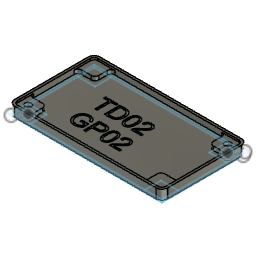
PDP_ETUDIANTS_3D_TD02_GP02 (Autodesk Fusion 360 archive; units mm, degrees)
design "Boitier Bas"
Autodesk Fusion 360 part; units mm, degrees
sketch "Sketch1" plane through (0, 0, 0) normal (0, 0, 1) x (1, 0, 0)
  line L0 (-40, 30) -> (39, 30)
  line L1 (39, 30) -> (39, -14)
  line L2 (39, -14) -> (-40, -14)
  line L3 (39, 30) -> (39, 28)
  line L4 (-40, 30) -> (-40, -14)
  circle A0 centre (-35, -9) radius 1.6
  circle A1 centre (34, 25) radius 1.6
  line L5 (39, 30) -> (37.8, 30)
  line L6 (-40, -14) -> (-38.8, -14)
  line L7 (37.8, 28.8) -> (-38.8, 28.8)
  line L8 (-38.8, 28.8) -> (-38.8, -12.8)
  line L9 (-38.8, -12.8) -> (37.8, -12.8)
  line L10 (37.8, -12.8) -> (37.8, 28.8)
  line L11 (-30.0372, -12.8) -> (-30.0372, -4.5)
  line L12 (-30.0372, -4.5) -> (-38.8, -4.5)
  line L13 (-30.037, 28.8) -> (-30.037, 20.5)
  line L14 (-30.037, 20.5) -> (-38.8, 20.5)
  line L15 (37.8, 20.5) -> (29.037, 20.5)
  line L16 (29.037, 20.5) -> (29.037, 28.8)
  line L17 (29.037, -12.8) -> (29.037, -4.5)
  line L18 (29.037, -4.5) -> (37.8, -4.5)
  line L19 (-31.8769, -9.5739) -> (-32.9414, -6.5822)
  line L20 (-32.9414, -6.5822) -> (-36.0646, -6.0083)
  line L21 (-36.0646, -6.0083) -> (-38.1231, -8.4261)
  line L22 (-38.1231, -8.4261) -> (-37.0586, -11.4178)
  line L23 (-37.0586, -11.4178) -> (-33.9354, -11.9917)
  line L24 (-33.9354, -11.9917) -> (-31.8769, -9.5739)
  line L25 (30.8264, 24.8932) -> (32.5057, 22.1982)
  line L26 (32.5057, 22.1982) -> (35.6793, 22.305)
  line L27 (35.6793, 22.305) -> (37.1736, 25.1068)
  line L28 (37.1736, 25.1068) -> (35.4943, 27.8018)
  line L29 (35.4943, 27.8018) -> (32.3207, 27.695)
  line L30 (32.3207, 27.695) -> (30.8264, 24.8932)
  point P0 (-35, -9)
  point P1 (34, 25)
  dimension "d1" = 79
  dimension "d2" = 44
  dimension "d6" = 3.2
  dimension "d8" = 3.2
  dimension "d32" = 8.3
  dimension "d33" = 8.763
  dimension "d35" = 8.763
  dimension "d36" = 8.763
  dimension "d37" = 8.3
  dimension "d38" = 8.3
  dimension "d39" = 8.3
  dimension "d65" = 2.75
  dimension "d70" = 2.75
  constraint horizontal L0
  constraint vertical L1
  constraint horizontal L2
  constraint perpendicular L0 L3
  constraint perpendicular L2 L4
  constraint perpendicular L3 L5
  constraint perpendicular L4 L6
  constraint horizontal L7
  constraint vertical L8
  constraint horizontal L9
  constraint vertical L10
  constraint coincident L9 L11.start
  constraint perpendicular L9 L11
  constraint coincident L8 L12.end
  constraint perpendicular L8 L12
  constraint coincident L7 L13.start
  constraint perpendicular L7 L13
  constraint coincident L8 L14.end
  constraint perpendicular L8 L14
  constraint coincident L10 L15.start
  constraint perpendicular L10 L15
  constraint coincident L7 L16.end
  constraint perpendicular L7 L16
  constraint coincident L9 L17.start
  constraint perpendicular L9 L17
  constraint coincident L10 L18.end
  constraint perpendicular L10 L18
  constraint coincident P0 A0.centre
  constraint coincident P1 A1.centre
  measures "d1" distance of L0.start L0.end
  measures "d2" distance of L0.start L2.end
  measures "d6" diameter of A0
  measures "d8" diameter of A1
  measures "d32" distance of L17.start L17.end
  measures "d33" distance of L13.end L14.end
  measures "d35" distance of L17.end L18.end
  measures "d36" distance of L15.start L15.end
  measures "d37" distance of L15.end L16.end
  measures "d38" distance of L11.start L11.end
  measures "d39" distance of L13.start L13.end
  measures "d65" distance of P0 L24
  measures "d70" distance of P1 L30
extrude "Extrude3" add sketch "Sketch1" along normal blind 5 contours L0 L1 L2 L3 L4 L5 L6
extrude "Extrude4" add sketch "Sketch1" along normal blind 4 contours L9 L10 L17 L18
extrude "Extrude5" add sketch "Sketch1" along normal blind 4 contours L7 L8 L13 L14
extrude "Extrude6" add sketch "Sketch1" along normal blind 4 contours A0 | L8 L9 L11 L12 | L19 L20 L21 L22 L23 L24
extrude "Extrude7" add sketch "Sketch1" along normal blind 4 contours A1 | L7 L10 L15 L16 | L25 L26 L27 L28 L29 L30
extrude "Extrude8" add sketch "Sketch1" along normal blind 2 contours L7 L8 L9 L10 L11 L12 L13 L14 L15 L16 L17 L18
extrude "Extrude9" cut sketch "Sketch1" along normal blind 2.4 contours L19 L20 L21 L22 L23 L24
extrude "Extrude10" cut sketch "Sketch1" along normal blind 4 contours A0
extrude "Extrude11" cut sketch "Sketch1" along normal blind 2.4 contours L25 L26 L27 L28 L29 L30
extrude "Extrude12" cut sketch "Sketch1" along normal blind 4.3 contours A1
form "Form1" [no effect]
fillet "Fillet1" radius 2 1 edges at (-38.8, 28.8, 4.5)
fillet "Fillet2" radius 3 1 edges at (-40, 30, 2.5)
fillet "Fillet3" radius 2 1 edges at (-38.8, -12.8, 4.5)
fillet "Fillet4" radius 3 1 edges at (-40, -14, 2.5)
fillet "Fillet5" radius 3 1 edges at (39, -14, 2.5)
fillet "Fillet6" radius 2 1 edges at (37.8, -12.8, 4.5)
fillet "Fillet7" radius 3 1 edges at (39, 30, 2.5)
fillet "Fillet8" radius 2 1 edges at (37.8, 28.8, 4.5)
sketch "Sketch3" plane through (0, 0, 2) normal (0, 0, 1) x (-1, 0, 0)
  line L0 (30.0372, 12.8) -> (-29.037, 12.8)
  line L1 (-29.037, 12.8) -> (-29.037, 4.5)
  line L2 (-29.037, 4.5) -> (-37.8, 4.5)
  line L3 (-37.8, 4.5) -> (-37.8, -20.5)
  line L4 (-37.8, -20.5) -> (-29.037, -20.5)
  line L5 (-29.037, -20.5) -> (-29.037, -28.8)
  line L6 (-29.037, -28.8) -> (30.037, -28.8)
  line L7 (30.037, -28.8) -> (30.037, -20.5)
  line L8 (30.037, -20.5) -> (38.8, -20.5)
  line L9 (38.8, -20.5) -> (38.8, 4.5)
  line L10 (38.8, 4.5) -> (30.0372, 4.5)
  line L11 (30.0372, 4.5) -> (30.0372, 12.8)
  line L12 (20.684, 3.5607) -> (-15.8059, 3.5607) construction
  line L13 (-15.8059, 3.5607) -> (-15.8059, -16.5576) construction
  line L14 (-15.8059, -16.5576) -> (20.684, -16.5576) construction
  line L15 (20.684, -16.5576) -> (20.684, 3.5607) construction
  dimension "d91" = 8
  text T0 "TD02 GP02" font "Arial" height 8 align left top in box 36.49 x 20.1184 at (20.684, 3.5607) x (-1, 0) y (0, -1) spacing 1 kerned
extrude "Extrude13" cut sketch "Sketch3" against normal blind 0.3 text T0
fillet "Fillet9" radius 2 1 edges at (-38.8, 20.5, 3)
fillet "Fillet10" radius 2 1 edges at (-30.037, 28.8, 3)
fillet "Fillet11" radius 2 1 edges at (-38.8, -4.5, 3)
fillet "Fillet12" radius 2 1 edges at (-30.0372, -12.8, 3)
fillet "Fillet13" radius 2 1 edges at (29.037, 28.8, 3)
fillet "Fillet14" radius 2 1 edges at (37.8, 20.5, 3)
fillet "Fillet15" radius 2 1 edges at (37.8, -4.5, 3)
fillet "Fillet16" radius 2 1 edges at (29.037, -12.8, 3)
fillet "Fillet17" radius 2 1 edges at (29.037, -4.5, 3)
fillet "Fillet18" radius 2 1 edges at (29.037, 20.5, 3)
fillet "Fillet19" radius 2 1 edges at (-30.037, 20.5, 3)
fillet "Fillet20" radius 2 1 edges at (-30.0372, -4.5, 3)
extrude "Extrude2" [suppressed]
sketch "Sketch2" plane through (0, 0, 0) normal (0, 1, 0) x (1, 0, 0)
  line L0 (-40, 0) -> (38.9993, 0)
  line L1 (38.9993, 0) -> (38.9993, -2.7)
  line L2 (-40, 0) -> (-40, -2.7)
  line L3 (-40, -2.7) -> (38.9993, -2.7)
  dimension "d27" = 2.7
  constraint horizontal L0
  constraint vertical L1
  constraint perpendicular L0 L2
  constraint perpendicular L1 L3
  measures "d27" distance of L0.start L2.end
